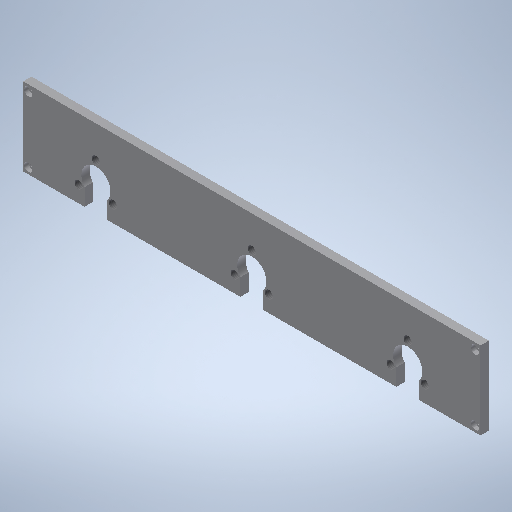
# Autodesk Inventor part: Top
Saved by Autodesk Inventor 2025 (Build 290162000, 162)
## iProperties
Created: 2010-12-14
Part Number: Top
Document SubType Name: Modeling
Designer: berny
Density: 2.71 g/cm^3
Material: Aluminum-6061
Mass: 542.356 g
Surface Area: 728.987 cm^2
Volume: 200.131 cm^3
Appearance: Aluminum - Flat
Author: berny
Autodesk Inventor part; units mm, degrees
ref_plane "YZ Plane" through (0, 0, 0) normal (1, 0, 0) x (0, 1, 0)
ref_plane "XZ Plane" through (0, 0, 0) normal (0, 1, 0) x (-1, 0, 0)
ref_plane "XY Plane" through (0, 0, 0) normal (0, 0, 1) x (1, 0, 0)
sketch "Sketch1" plane through (0, 0, 0) normal (0, 0, 1) x (1, 0, 0)
  line L0 (0, 0) -> (440, 0)
  line L1 (440, 0) -> (440, 75)
  line L2 (440, 75) -> (0, 75)
  line L3 (0, 75) -> (0, 0)
  dimension "d0" = 75
  dimension "d1" = 440
  constraints: 8 end point, 2 parallel, 1 horizontal, 1 perpendicular
  measures "d0" distance of L2.end L0.start
  measures "d1" distance between parallel lines of L1 L3
extrude "Extrusion1" add sketch "Sketch1" along normal blind 8
sketch "Sketch2" plane through (0, 0, 8) normal (0, 0, 1) x (1, 0, 0)
  line L0 (0, 0) -> (0, 75) projected
  line L1 (440, 0) -> (0, 0) projected
  circle A0 centre (70, 25) radius 14
  line L2 (59, 16.3397) -> (59, 0)
  line L3 (81, 16.3397) -> (81, 0)
  circle A1 centre (220, 25) radius 14
  line L4 (209, 16.3397) -> (209, 0)
  line L5 (231, 16.3397) -> (231, 0)
  circle A2 centre (370, 25) radius 14
  line L6 (359, 16.3397) -> (359, 0)
  line L7 (381, 16.3397) -> (381, 0)
  line L8 (209, 0) -> (231, 0)
  line L9 (359, 0) -> (381, 0)
  line L10 (521.97, 0) -> (544.83, 0)
  line L11 (671.8667, 0) -> (697.23, 0)
  line L12 (826.77, 0) -> (849.63, 0)
  line L13 (674.37, 0) -> (697.23, 0)
  dimension "d4" = 22
  dimension "d5" = 11
  dimension "d7" = 25
  dimension "d8" = 28
  dimension "d9" = 70
  dimension "d17" = 150
  dimension "d58" = 440
  constraints: 24 end point, 6 collinear, 6 point on circle, 3 centre point, 3 point on line, 2 perpendicular, 1 horizontal, 16 other
  measures "d4" distance between parallel lines of L3 L2
  measures "d5" distance from line of L2 A0.centre
  measures "d7" distance from line of L1 A0.centre
  measures "d8" diameter of A0
  measures "d9" distance from line of L0 A0.centre
  measures "d17" distance of A0.centre A1.centre
  measures "d58" distance of L1.start L0.start
extrude "Extrusion4" cut sketch "Sketch2" against normal up to next
sketch "Sketch3" plane through (0, 0, 8) normal (0, 0, 1) x (1, 0, 0)
  arc A0 (81, 16.3397) -> (59, 16.3397) centre (70, 25) ccw projected
  circle A1 centre (70, 25) radius 19
  line L0 (209, 0) -> (81, 0) projected
  point P0 (70, 44)
  point P1 (53.5455, 15.5)
  point P2 (86.4545, 15.5)
  point P3 (220, 44)
  point P4 (236.4545, 15.5)
  point P5 (203.5455, 15.5)
  point P6 (370, 44)
  point P7 (386.4545, 15.5)
  point P8 (353.5455, 15.5)
  dimension "d59" = 38
  dimension "d62" = 360
  dimension "d66" = 150
  constraints: 2 vertical alignment, 1 coincident, 1 horizontal, 12 other
  measures "d66" distance of point (70, 44) point (220, 44)
hole "Hole1" at (70, 44, 8) at (86.4545, 15.5, 8) at (53.5455, 15.5, 8) at (203.5455, 15.5, 8) at (236.4545, 15.5, 8) at (220, 44, 8) at (353.5455, 15.5, 8) at (370, 44, 8) at (386.4545, 15.5, 8) direction (0, 0, -1) diameter 7.7978 end through all thread size "3/8-16 UNC" class "2B" standard "ANSI Unified Screw Threads"
sketch "Sketch4" plane through (0, 0, 8) normal (0, 0, 1) x (1, 0, 0)
  line L0 (440, 75) -> (440, 0) projected
  line L1 (0, 0) -> (0, 75) projected
  line L2 (440, 0) -> (0, 0) projected
  point P0 (59, 0)
  point P1 (5, 69)
  point P2 (5, 6)
  point P3 (435, 6)
  point P4 (435, 69)
  dimension "d42" = 6
  dimension "d44" = 5
  dimension "d45" = 5
  dimension "d71" = 69
  constraints: 2 horizontal alignment, 2 vertical alignment
  measures "d42" distance from line of L2 point (5, 6)
  measures "d44" distance from line of L0 point (435, 69)
  measures "d45" distance from line of L1 point (5, 69)
  measures "d71" distance from line of L2 point (5, 69)
hole "Hole2" at (5, 69, 8) at (5, 6, 8) at (435, 6, 8) at (435, 69, 8) direction (0, 0, -1) diameter 4.5 end through all counterbore diameter 8 counterbore depth 4 clearance for "Socket Head Cap Screw" size "M4" standard "Ansi Metric M Profile"
equation "\"d4\" = 2 * d5"
equation "\"d9\" = -d17 + 0.5 * d58"
equation "\"d44\" = d45"
body "Solid1"
